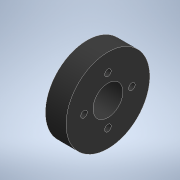
# Autodesk Inventor part: Pulley - VBelt (2.5in OD)
Saved by Autodesk Inventor 2022.1 (Build 261234020, 234B)
## iProperties
Created: 2022-04-06
Part Number: Pulley - VBelt (2.5in OD)
Material: Nylon 6/6
Document SubType Name: Modeling
Designer: NCai2
Density: 1.13 g/cm^3
Appearance: Rubber - Black
Mass: 27.9154 g
Surface Area: 87.8625 cm^2
Volume: 24.7039 cm^3
Author: NCai2
Autodesk Inventor part; units mm, degrees
ref_plane "YZ Plane" through (0, 0, 0) normal (1, 0, 0) x (0, 1, 0)
ref_plane "XZ Plane" through (0, 0, 0) normal (0, 1, 0) x (-1, 0, 0)
ref_plane "XY Plane" through (0, 0, 0) normal (0, 0, 1) x (1, 0, 0)
sketch "Sketch1" plane through (0, 0, 0) normal (0, 0, 1) x (1, 0, 0)
  line L0 (0, 0) -> (4.7625, 0) construction
  line L1 (4.7625, 0) -> (4.7625, 22.225)
  line L2 (4.7625, 22.225) -> (0, 22.225)
  line L3 (0, 22.225) -> (0, 0)
  line L4 (3.3, 22.225) -> (1.4923, 16.975)
  line L5 (1.4923, 16.975) -> (0, 16.975)
  line L6 (0, 7.9375) -> (4.7625, 7.9375)
  line L7 (0, 0) -> (-4.7625, 0) construction
  line L8 (-4.7625, 0) -> (-4.7625, 22.225)
  line L9 (-4.7625, 22.225) -> (0, 22.225)
  line L10 (-3.3, 22.225) -> (-1.4923, 16.975)
  line L11 (-1.4923, 16.975) -> (0, 16.975)
  line L12 (0, 7.9375) -> (-4.7625, 7.9375)
  dimension "d0" = 4.7625
  dimension "d1" = 22.225
  dimension "d2" = 19
  dimension "d3" = 3.3
  dimension "d4" = 5.25
  dimension "d5" = 7.9375
  constraints: 26 end point, 6 point on line, 5 symmetric about line, 3 perpendicular, 2 parallel, 1 horizontal
  measures "d0" distance of L2.end L1.end
  measures "d1" distance of L1.end L0.end
  measures "d2" angle of L3 L4
  measures "d3" distance of L2.end L4.start
  measures "d4" distance between parallel lines of L2 L5
  measures "d5" distance between parallel lines of L0 L6
revolve "Revolution1" add sketch "Sketch1" angle 360 about axis through (0, 0, 0) along (-1, 0, 0) contours L6 L3 L5 L4 L2 L1 | L12 L8 L9 L10 L11 L3
sketch "Sketch2" plane through (4.7625, 0, 0) normal (1, 0, 0) x (0, 0, -1)
  circle A0 centre (0, 0) radius 12.7 construction
  circle A1 centre (0, 12.7) radius 1.7272
  circle A2 centre (-12.7, 0) radius 1.7272
  circle A3 centre (0, -12.7) radius 1.7272
  circle A4 centre (12.7, 0) radius 1.7272
  dimension "d7" = 25.4
  dimension "d8" = 3.4544
  dimension "d11" = 360
  constraints: 4 centre point, 1 coincident, 1 vertical alignment, 11 other
  measures "d8" diameter of A1
extrude "Extrusion1" cut sketch "Sketch2" against normal through all
sketch "Sketch3" plane through (-4.7625, 0, 0) normal (-1, 0, 0) x (0, 0, 1)
  circle A0 centre (0, 0) radius 15.875
  dimension "d15" = 31.75
  constraints: 1 centre point, 1 coincident
  measures "d15" diameter of A0
extrude "Extrusion2" cut sketch "Sketch3" against normal blind 3.175
thicken "Thicken1" operation add thickness 9.525 both sides no extend neighbours yes toward (1, 0, 0) faces at (4.7625, 11.759, 7.2429)
chamfer "Chamfer1" distance 1.5875 angle 45 1 edges at (-1.5875, 0, -15.875)
body "Solid1"
